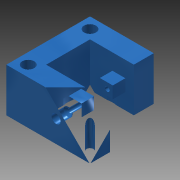
# Autodesk Inventor part: Infill3DBody
Saved by Autodesk Inventor 2015 SP1 (Build 190203100, 203)
## iProperties
Created: 2015-04-27
Part Number: Infill3DBody
Material: Generic
Document SubType Name: Modeling
Designer: Jack
Density: 1 g/cm^3
Appearance: Cyan
Author: Jack
Autodesk Inventor part; units mm, degrees
ref_plane "YZ Plane" through (0, 0, 0) normal (1, 0, 0) x (0, 1, 0)
ref_plane "XZ Plane" through (0, 0, 0) normal (0, 1, 0) x (-1, 0, 0)
ref_plane "XY Plane" through (0, 0, 0) normal (0, 0, 1) x (1, 0, 0)
sketch "Sketch1" plane through (0, 0, 0) normal (0, 0, 1) x (1, 0, 0)
  line L0 (42, 0) -> (0, 0)
  line L1 (0, 0) -> (0, 42)
  line L2 (0, 42) -> (42, 42)
  line L3 (42, 42) -> (42, 0)
  dimension "d3" = 42
  dimension "d4" = 42
  constraints: 8 end point, 2 parallel, 1 coincident, 1 horizontal, 1 perpendicular
  measures "d3" distance of L1.end L2.end
  measures "d4" distance of L0.end L1.end
extrude "Extrusion1" add sketch "Sketch1" along normal blind 22
sketch "Sketch2" plane through (0, 0, 22) normal (0, 0, 1) x (1, 0, 0)
  line L0 (0, 0) -> (42, 0) projected
  line L1 (0, 42) -> (0, 0) projected
  point P0 (5.5, 36.5)
  point P1 (5.5, 5.5)
  point P2 (36.5, 5.5)
  dimension "d9" = 31
  dimension "d10" = 31
  dimension "d11" = 5.5
  dimension "d12" = 5.5
  constraints: 1 horizontal alignment, 1 vertical alignment
  measures "d9" distance of point (5.5, 36.5) point (5.5, 5.5)
  measures "d10" distance of point (36.5, 5.5) point (5.5, 5.5)
  measures "d11" distance from line of L0 point (36.5, 5.5)
  measures "d12" distance from line of L1 point (5.5, 5.5)
hole "Hole1" at (5.5, 36.5, 22) at (5.5, 5.5, 22) direction (0, 0, -1) diameter 3.5 end through all counterbore diameter 6 counterbore depth 16
sketch "Sketch3" plane through (0, 0, 22) normal (0, 0, 1) x (1, 0, 0)
  line L0 (0, 0) -> (42, 0) projected
  line L1 (42, 42) -> (0, 42) projected
  line L2 (0, 42) -> (0, 0) projected
  line L3 (42, 42) -> (42, 0) projected
  line L4 (42, 32) -> (10, 32)
  line L5 (10, 32) -> (10, 10)
  line L6 (10, 10) -> (42, 10)
  dimension "d20" = 10
  dimension "d21" = 10
  dimension "d22" = 10
  constraints: 6 end point, 2 point on line, 1 horizontal, 1 perpendicular, 1 vertical
  measures "d20" distance between parallel lines of L0 L6
  measures "d21" distance between parallel lines of L2 L5
  measures "d22" distance between parallel lines of L1 L4
extrude "Extrusion2" cut sketch "Sketch3" against normal up to next contours L6 L5 L4 L3
sketch "Sketch4" plane through (42, 42, 22) normal (1, 0, 0) x (0, 0, -1)
  line L0 (0, -10) -> (22, -10) projected
  line L1 (22, 0) -> (22, -10) projected
  line L2 (22, 0) -> (0, 0) projected
  line L3 (0, -10) -> (0, 0) projected
extrude "Extrusion3" cut sketch "Sketch4" against normal blind 10
ref_plane "Work Plane1" through (24.5, 0, 0) normal (-1, 0, 0) x (0, 0, 1)
sketch "Sketch7" plane through (24.5, 0, 0) normal (-1, 0, 0) x (0, 0, 1)
  line L0 (0, 10) -> (22, 10) projected
  line L1 (14, 10) -> (14, 16.3)
  line L2 (14, 16.3) -> (8, 16.3)
  line L3 (8, 16.3) -> (8, 10)
  line L4 (0, 10) -> (0, 0) projected
  dimension "d45" = 6
  dimension "d46" = 8
  dimension "d47" = 6.3
  constraints: 6 end point, 2 perpendicular, 2 point on line, 1 vertical
  measures "d45" distance of L1.end L2.end
  measures "d46" distance between parallel lines of L4 L3
  measures "d47" distance of L1.start L1.end
extrude "Extrusion4" add sketch "Sketch7" along normal mid plane 6.5
ref_plane "Work Plane2" through (24.5, 0, 0) normal (-1, 0, 0) x (0, 0, 1)
sketch "Sketch8" plane through (24.5, 0, 0) normal (-1, 0, 0) x (0, 0, 1)
  line L0 (0, 32) -> (22, 32) projected
  line L1 (14, 32) -> (14, 25.7)
  line L2 (14, 25.7) -> (8, 25.7)
  line L3 (8, 25.7) -> (8, 32)
  line L4 (22, 32) -> (22, 42) projected
  point P0 (0, 0)
  dimension "d51" = 6
  dimension "d52" = 6.3
  dimension "d53" = 8
  constraints: 6 end point, 2 perpendicular, 2 point on line, 1 vertical
  measures "d51" distance of L1.end L2.end
  measures "d52" distance of L2.end L3.end
  measures "d53" distance between parallel lines of L4 L1
extrude "Extrusion5" add sketch "Sketch8" along normal mid plane 6.5
sketch "Sketch5" plane through (0, 42, 22) normal (0, 1, 0) x (1, 0, 0)
  line L0 (0, 22) -> (32, 22) projected
  line L1 (0, 22) -> (0, 0) projected
  point P0 (25, 11)
  dimension "d27" = 11
  dimension "d29" = 25
  measures "d27" distance from line of L0 point (25, 11)
  measures "d29" distance from line of L1 point (25, 11)
hole "Hole2" at (25, 42, 11) direction (0, -1, 0) diameter 2.3 end through all
sketch "Sketch6" plane through (0, 0, 0) normal (0, -1, 0) x (1, 0, 0)
  circle A0 centre (25, 11) radius 1.15 projected
hole "Hole3" at (25, 0, 11) direction (0, 1, 0) diameter 4.5 depth 6 tip angle 90
sketch "Sketch9" plane through (0, 42, 22) normal (0, 1, 0) x (1, 0, 0)
  circle A0 centre (25, 11) radius 1.15 projected
hole "Hole4" at (25, 42, 11) direction (0, -1, 0) diameter 12.4 depth 7
sketch "Sketch10" plane through (0, 0, 0) normal (0, 0, -1) x (-1, 0, 0)
  line L0 (-10, 32) -> (-10, 10) projected
  line L1 (-10, 10) -> (-42, 10) projected
  circle A0 centre (-21, 21) radius 11.25
  dimension "d63" = 11
  dimension "d64" = 11
  dimension "d65" = 22.5
  constraints: 1 centre point, 1 coincident
  measures "d63" distance from line of L1 point (-21, 21)
  measures "d64" distance from line of L0 point (-21, 21)
  measures "d65" diameter of A0
extrude "Extrusion6" cut sketch "Sketch10" against normal blind 3 contours A0 L0 | L0 A0 L1 | L1 A0 picked at (-18.1333, 21.9679)
sketch "Sketch11" plane through (0, 0, 22) normal (0, 0, 1) x (1, 0, 0)
  circle A0 centre (5.5, 5.5) radius 3 projected
  point P0 (36.5, 5.5)
  dimension "d69" = 31
  constraints: 1 horizontal alignment
  measures "d69" distance of A0.centre point (36.5, 5.5)
hole "Hole5" at (36.5, 5.5, 22) direction (0, 0, -1) diameter 3.5 end through all
sketch "Sketch13" plane through (42, 0, 22) normal (1, 0, 0) x (0, 0, -1)
  line L0 (22, 10) -> (0, 10) projected
  line L1 (22, 0) -> (0, 0) projected
  line L2 (22, 10) -> (22, 0) projected
  line L3 (4, 10) -> (4, 0)
  line L4 (18, 0) -> (18, 10)
  dimension "d83" = 14
  dimension "d84" = 4
  constraints: 4 end point, 4 point on line, 2 perpendicular
  measures "d83" distance between parallel lines of L4 L3
  measures "d84" distance between parallel lines of L2 L4
extrude "Extrusion8" cut sketch "Sketch13" against normal blind 10 contours L4 L1 L3 L0
sketch "Sketch12" plane through (0, 0, 0) normal (0, -1, 0) x (1, 0, 0)
  line L0 (42, 0) -> (0, 0) projected
  line L1 (0, 22) -> (42, 22) projected
  line L2 (0, 0) -> (0, 22) projected
  line L3 (0, 5.7321) -> (3, 4)
  line L4 (3, 4) -> (3, 18)
  line L5 (3, 18) -> (0, 16.2679)
  dimension "d77" = 3
  dimension "d78" = 60
  dimension "d79" = 4
  dimension "d80" = 4
  constraints: 6 end point, 2 point on line, 1 equal length, 1 vertical
  measures "d77" distance between parallel lines of L2 L4
  measures "d78" angle of L2 L5
  measures "d79" distance from line of L1 L4.end
  measures "d80" distance from line of L0 L3.end
body "Solid1"
